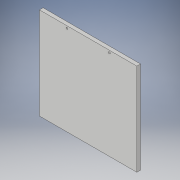
# Autodesk Inventor part: new side wall
Saved by Autodesk Inventor 2019 (Build 230136000, 136)
## iProperties
Created: 2020-03-01
Part Number: new side wall
Material: Generic
Document SubType Name: Modeling
Designer: KiranM
Density: 1 g/cm^3
Appearance: Default
Author: KiranM
Autodesk Inventor part; units mm, degrees
ref_plane "YZ Plane" through (0, 0, 0) normal (1, 0, 0) x (0, 1, 0)
ref_plane "XZ Plane" through (0, 0, 0) normal (0, 1, 0) x (-1, 0, 0)
ref_plane "XY Plane" through (0, 0, 0) normal (0, 0, 1) x (1, 0, 0)
sketch "Sketch1" plane through (0, 0, 0) normal (0, 0, 1) x (1, 0, 0)
  line L0 (0, 0) -> (265, 0)
  line L1 (265, 0) -> (265, -250)
  line L2 (265, -250) -> (0, -250)
  line L3 (0, -250) -> (0, 0)
  line L4 (0, 0) -> (0, -6)
  circle A0 centre (75, -6) radius 2.5
  line L5 (265, 0) -> (265, -6)
  circle A1 centre (190, -6) radius 2.5
  constraints: 12 end point, 2 centre point, 2 parallel, 2 point on line, 1 horizontal, 1 perpendicular
extrude "Extrusion1" add sketch "Sketch1" along normal blind 10
body "Solid1"
